Autodesk Inventor part; units mm, degrees
(part 2 of 2)
  spline S158 degree 2 poles (-13.3047, -14.1269) (-13.2533, -14.0704) (-13.1095, -13.8957) (-13.0401, -13.7698) knots 0 0 0 1 2 2 2
  spline S159 degree 2 poles (-13.0401, -13.7698) (-12.9733, -13.6491) (-12.8885, -13.3639) (-12.8885, -13.179) knots 0 0 0 1 2 2 2
  spline S160 degree 2 poles (-12.8885, -13.179) (-12.8885, -12.976) (-13.0555, -12.6138) (-13.2148, -12.4777) knots 0 0 0 1 2 2 2
  spline S161 degree 2 poles (-13.2148, -12.4777) (-13.3766, -12.3441) (-13.8673, -12.1951) (-14.173, -12.1951) knots 0 0 0 1 2 2 2
  spline S162 degree 2 poles (-14.173, -12.1951) (-14.4992, -12.1951) (-14.9693, -12.3518) (-15.1312, -12.488) knots 0 0 0 1 2 2 2
  spline S163 degree 2 poles (-15.1312, -12.488) (-15.2879, -12.6215) (-15.4471, -12.9786) (-15.4471, -13.179) knots 0 0 0 1 2 2 2
  spline S164 degree 2 poles (-15.4471, -13.179) (-15.4471, -13.3614) (-15.3572, -13.6722) (-15.2904, -13.7929) knots 0 0 0 1 2 2 2
  spline S165 degree 2 poles (-15.2904, -13.7929) (-15.2236, -13.9085) (-15.0849, -14.0807) (-15.0361, -14.1295) knots 0 0 0 1 2 2 2
  line L273 (-15.0361, -14.1295) -> (-15.0361, -14.1603)
  line L274 (-15.0361, -14.1603) -> (-15.5396, -14.1603)
  spline S166 degree 2 poles (-15.5396, -14.1603) (-15.5884, -14.055) (-15.6783, -13.87) (-15.7194, -13.739) knots 0 0 0 1 2 2 2
  spline S167 degree 2 poles (-15.7194, -13.739) (-15.7657, -13.6003) (-15.8119, -13.3639) (-15.8119, -13.1738) knots 0 0 0 1 2 2 2
  spline S168 degree 2 poles (-12.9476, -16.796) (-13.1583, -16.9758) (-13.7748, -17.1762) (-14.1704, -17.1762) knots 0 0 0 1 2 2 2
  spline S169 degree 2 poles (-14.1704, -17.1762) (-14.5557, -17.1762) (-15.18, -16.9809) (-15.3906, -16.796) knots 0 0 0 1 2 2 2
  spline S170 degree 2 poles (-15.3906, -16.796) (-15.6115, -16.6007) (-15.8222, -16.0844) (-15.8222, -15.7735) knots 0 0 0 1 2 2 2
  spline S171 degree 2 poles (-15.8222, -15.7735) (-15.8222, -15.4524) (-15.6038, -14.9387) (-15.3906, -14.7511) knots 0 0 0 1 2 2 2
  spline S172 degree 2 poles (-15.3906, -14.7511) (-15.18, -14.5687) (-14.5609, -14.3735) (-14.1704, -14.3735) knots 0 0 0 1 2 2 2
  spline S173 degree 2 poles (-14.1704, -14.3735) (-13.7722, -14.3735) (-13.166, -14.5713) (-12.9476, -14.7537) knots 0 0 0 1 2 2 2
  spline S174 degree 2 poles (-12.9476, -14.7537) (-12.737, -14.9387) (-12.5186, -15.455) (-12.5186, -15.7735) knots 0 0 0 1 2 2 2
  spline S175 degree 2 poles (-12.5186, -15.7735) (-12.5186, -16.0972) (-12.7447, -16.6161) (-12.9476, -16.796) knots 0 0 0 1 2 2 2
  spline S176 degree 2 poles (-14.1704, -16.7369) (-13.857, -16.7369) (-13.3715, -16.6007) (-13.2122, -16.4774) knots 0 0 0 1 2 2 2
  spline S177 degree 2 poles (-13.2122, -16.4774) (-13.0478, -16.3515) (-12.8834, -15.997) (-12.8834, -15.7761) knots 0 0 0 1 2 2 2
  spline S178 degree 2 poles (-12.8834, -15.7761) (-12.8834, -15.5475) (-13.0427, -15.2033) (-13.2122, -15.0722) knots 0 0 0 1 2 2 2
  spline S179 degree 2 poles (-13.2122, -15.0722) (-13.374, -14.9464) (-13.8621, -14.8128) (-14.1704, -14.8128) knots 0 0 0 1 2 2 2
  spline S180 degree 2 poles (-14.1704, -14.8128) (-14.7946, -14.8128) (-15.4574, -15.3368) (-15.4574, -15.7761) knots 0 0 0 1 2 2 2
  spline S181 degree 2 poles (-15.4574, -15.7761) (-15.4574, -16.2154) (-14.7946, -16.7369) (-14.1704, -16.7369) knots 0 0 0 1 2 2 2
  line L275 (-15.7554, -20.3564) -> (-15.7554, -19.9351)
  line L276 (-15.7554, -19.9351) -> (-13.0247, -19.9351)
  line L277 (-13.0247, -19.9351) -> (-14.882, -19.108)
  line L278 (-14.882, -19.108) -> (-14.882, -18.8511)
  line L279 (-14.882, -18.8511) -> (-13.0247, -18.0316)
  line L280 (-13.0247, -18.0316) -> (-15.7554, -18.0316)
  line L281 (-15.7554, -18.0316) -> (-15.7554, -17.6386)
  line L282 (-15.7554, -17.6386) -> (-12.5854, -17.6386)
  line L283 (-12.5854, -17.6386) -> (-12.5854, -18.214)
  line L284 (-12.5854, -18.214) -> (-14.3502, -19.0052)
  line L285 (-14.3502, -19.0052) -> (-12.5854, -19.7707)
  line L286 (-12.5854, -19.7707) -> (-12.5854, -20.3564)
  line L287 (-12.5854, -20.3564) -> (-15.7554, -20.3564)
  point P0 (0, 0)
  constraints: 2 other
extrude "Extrusion8" add sketch "Sketch9" along normal blind 0.5
sketch "Sketch10" plane through (0, 2, 0) normal (0, 1, 0) x (1, 0, 0)
  line L0 (29.0932, 58.6501) -> (-22.9068, 58.6501) projected
  line L1 (-22.9068, 58.6501) -> (-17.9068, 58.6501)
  line L2 (-22.9068, 58.6501) -> (-22.9068, 53.6501)
  line L3 (-22.9068, 58.6501) -> (-22.9068, -60.3499) projected
  line L4 (-22.9068, 53.6501) -> (-17.9068, 58.6501)
  line L5 (-17.9068, 58.6501) -> (-15.9068, 58.6501)
  line L6 (-15.9068, 58.6501) -> (-22.9068, 51.6501)
  line L7 (-22.9068, 51.6501) -> (-22.9068, 46.6501)
  line L8 (-22.9068, 46.6501) -> (-10.9068, 58.6501)
  line L9 (-10.9068, 58.6501) -> (-8.9068, 58.6501)
  line L10 (-8.9068, 58.6501) -> (-22.9068, 44.6501)
  line L11 (-22.9068, 44.6501) -> (-22.9068, 39.6501)
  line L12 (-22.9068, 39.6501) -> (-3.9068, 58.6501)
  line L13 (-3.9068, 58.6501) -> (-1.9068, 58.6501)
  line L14 (-1.9068, 58.6501) -> (-22.9068, 37.6501)
  point P0 (0, 0)
  dimension "d36" = 5
  dimension "d37" = 5
  dimension "d38" = 2
  dimension "d39" = 5
  dimension "d40" = 2
  dimension "d41" = 5
  dimension "d42" = 2
  constraints: 26 end point, 12 point on line, 2 parallel
  measures "d36" distance of L0.end L1.end
  measures "d37" distance of L0.end L2.end
  measures "d38" distance of L1.end L5.end
  measures "d39" distance of L6.end L7.end
  measures "d40" distance of L8.end L9.end
  measures "d41" distance of L10.end L11.end
  measures "d42" distance of L12.end L13.end
extrude "Extrusion9" cut sketch "Sketch10" against normal blind 0.5 contours L14 L3 L12 L0 | L10 L3 L8 L0 | L6 L3 L4 L0
equation "\"BendRadius\" = Thickness"
equation "\"BendReliefWidth\" = Thickness"
equation "\"BendReliefDepth\" = 0.5 * Thickness"
equation "\"CornerReliefSize\" = 4 * Thickness"
equation "\"MinimumRemnant\" = 2 * Thickness"
equation "\"TransitionRadius\" = BendRadius"
equation "\"JacobiRadiusSize\" = BendRadius"
equation "\"GapSize\" = Thickness"
equation "\"Thickness\" = 0.5"
body "Solid1"
